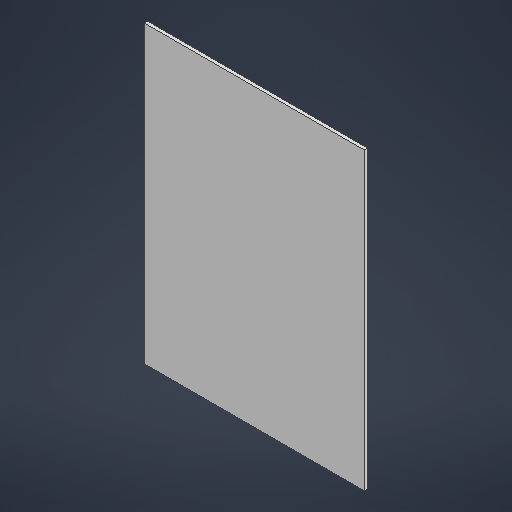
# Autodesk Inventor part: plane
Saved by Autodesk Inventor 2027 (Build 310192060, 192F)
## iProperties
Created: 2026-06-14
Part Number: plane
Material: Ogólny
Document SubType Name: Modeling
Designer: User
Density: 1 g/cm^3
Appearance: Domyślna
Author: User
Autodesk Inventor part; units mm, degrees
ref_plane "YZ Plane" through (0, 0, 0) normal (1, 0, 0) x (0, 1, 0)
ref_plane "XZ Plane" through (0, 0, 0) normal (0, 1, 0) x (-1, 0, 0)
ref_plane "XY Plane" through (0, 0, 0) normal (0, 0, 1) x (1, 0, 0)
sketch "Szkic1" plane through (0, 0, 0) normal (0, 1, 0) x (-1, 0, 0)
  line L0 (33.5, -0.5) -> (-33.5, -0.5)
  line L1 (-33.5, -0.5) -> (-33.5, 0.5)
  line L2 (-33.5, 0.5) -> (33.5, 0.5)
  line L3 (33.5, 0.5) -> (33.5, -0.5)
  line L4 (33.5, -0.5) -> (-33.5, 0.5) construction
  line L5 (-33.5, -0.5) -> (33.5, 0.5) construction
  point P0 (0, 0)
  dimension "d0" = 67
  dimension "d1" = 1
  constraints: 12 end point, 2 midpoint, 2 parallel, 1 horizontal, 1 perpendicular
  measures "d0" distance of L1.end L2.end
  measures "d1" distance of L0.end L1.end
extrude "Wyciągnięcie proste1" add sketch "Szkic1" along normal blind 90
